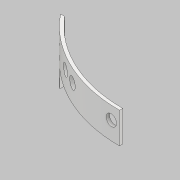
# Autodesk Inventor part: CW006
Saved by Autodesk Inventor 2017 (Build 210142000, 142)
## iProperties
Created: 2017-05-25
Part Number: CW006
Material: ABS Plastic
Document SubType Name: Modeling
Designer: zallen
Density: 1.06 g/cm^3
Appearance: CR White
Author: zallen
Autodesk Inventor part; units mm, degrees
sketch "Sketch1" plane through (0, 0, 0) normal (0, 0, 1) x (1, 0, 0)
  circle A0 centre (0, 225) radius 225 construction
  line L0 (0, 0) -> (0, 5)
  arc A1 (-168.523, 83.5786) -> (0, 5) centre (0, 225) ccw
  arc A2 (-175, 83.5786) -> (0, 0) centre (0, 225) ccw
  line L1 (-175, 83.5786) -> (-168.523, 83.5786)
  line L2 (-175, 83.5786) -> (-168.523, 83.5786) construction
  dimension "d0" = 450
  dimension "d3" = 175
  dimension "d6" = 0
  dimension "d18" = 5
  constraints: 7 point on circle, 6 end point, 3 centre point, 2 concentric, 1 collinear, 1 horizontal, 1 vertical, 1 vertical alignment
  measures "d0" diameter of A0
  measures "d3" horizontal distance of L0.start L1.start
  measures "d6" distance between parallel lines of L2 L1
  measures "d18" distance of L0.start L0.end
extrude "Extrusion1" add sketch "Sketch1" along normal blind 75
sketch "Sketch2" plane through (0, 0, 0) normal (0, 1, 0) x (-1, 0, 0)
  line L0 (0, 0) -> (150, 0)
  line L1 (150, 0) -> (150, 27)
  line L2 (150, 27) -> (0, 27)
  line L3 (0, 27) -> (0, 0)
  line L4 (175, 0) -> (175, 75) projected
  dimension "d7" = 27
  dimension "d8" = 25
  constraints: 8 end point, 2 parallel, 1 horizontal, 1 perpendicular
  measures "d7" distance of L1.end L0.end
  measures "d8" distance between parallel lines of L1 L4
extrude "Extrusion2" cut sketch "Sketch2" along normal through all
ref_plane "Work Plane1" through (-175, 83.5786, 0) normal (-0.7778, -0.6285, 0) x (0.6285, -0.7778, 0)
sketch "Sketch3" plane through (-175, 83.5786, 0) normal (-0.7778, -0.6285, 0) x (0.6285, -0.7778, 0)
  circle A0 centre (16, 47.5) radius 3
  circle A1 centre (16, 27.5) radius 3
  line L0 (0, 0) -> (0, 75) projected
  line L1 (36.1564, 0) -> (0, 0) projected
  point P0 (175, 0)
  dimension "d11" = 6
  dimension "d12" = 6
  dimension "d13" = 16
  dimension "d14" = 27.5
  dimension "d15" = 20
  constraints: 2 centre point, 1 vertical alignment
  measures "d11" diameter of A0
  measures "d12" diameter of A1
  measures "d13" distance from line of L0 A1.centre
  measures "d14" distance from line of L1 A1.centre
  measures "d15" distance of A0.centre A1.centre
extrude "Extrusion3" cut sketch "Sketch3" along normal through all both and the other way through all
ref_plane "Work Plane2" through (-175, 83.5786, 75) normal (0.431, 0.9024, 0) x (0.9024, -0.431, 0)
sketch "Sketch4" plane through (-175, 83.5786, 75) normal (0.431, 0.9024, 0) x (0.9024, -0.431, 0)
  circle A0 centre (75, 20) radius 8.5
  circle A1 centre (101, 20) radius 8.5
  point P0 (193.934, 75)
  point P1 (0, 0)
  point P2 (193.934, 0)
  dimension "d19" = 17
  dimension "d20" = 17
  dimension "d21" = 26
  dimension "d22" = 75
  dimension "d23" = 20
  constraints: 2 centre point, 1 horizontal alignment
  measures "d19" diameter of A0
  measures "d20" diameter of A1
  measures "d21" distance of A1.centre A0.centre
  measures "d22" horizontal distance of point (0, 0) A0.centre
  measures "d23" vertical distance of point (0, 0) A0.centre
extrude "Extrusion4" cut sketch "Sketch4" along normal through all both and the other way through all
ref_plane "Work Plane3" through (0, 0, 0) normal (0, -1, 0) x (1, 0, 0)
sketch "Sketch5" plane through (0, 0, 0) normal (0, -1, 0) x (1, 0, 0)
  circle A0 centre (-13, 55) radius 8.5
  line L0 (0, 75) -> (-175, 75) projected
  line L1 (0, 27) -> (0, 75) projected
  point P0 (0, 0)
  dimension "d26" = 17
  dimension "d27" = 20
  dimension "d28" = 13
  constraints: 1 centre point
  measures "d26" diameter of A0
  measures "d27" distance from line of A0.centre L0
  measures "d28" distance from line of L1 A0.centre
extrude "Extrusion5" cut sketch "Sketch5" against normal through all
body "Solid1"
